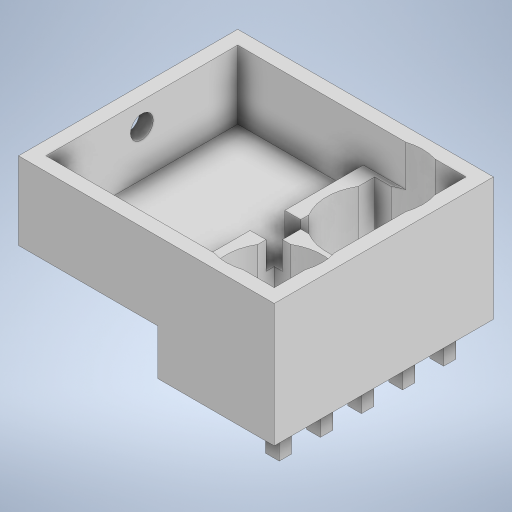
# Autodesk Inventor part: Suporte Eletroimã
Saved by Autodesk Inventor 2023 (Build 270158000, 158)
## iProperties
Created: 2023-03-07
Part Number: Suporte Eletroimã
Material: Genérico
Document SubType Name: Modeling
Designer: Inteli
Density: 1 g/cm^3
Appearance: Padrão
Author: Inteli
## iProperties of the stored document Suporte Eletroimã_3DPrint.ipt
Created: 2023-03-09
Part Number: Suporte Eletroimã_3DPrint
Material: Genérico
Document SubType Name: Modeling
Designer: Inteli
Density: 1 g/cm^3
Appearance: Padrão
Author: Inteli
Autodesk Inventor part; units mm, degrees
ref_plane "YZ Plane" through (0, 0, 0) normal (1, 0, 0) x (0, 1, 0)
ref_plane "XZ Plane" through (0, 0, 0) normal (0, 1, 0) x (-1, 0, 0)
ref_plane "XY Plane" through (0, 0, 0) normal (0, 0, 1) x (1, 0, 0)
sketch "Esboço1" plane through (0, 0, 0) normal (0, 1, 0) x (-1, 0, 0)
  circle A0 centre (0, 11) radius 10.5
  circle A1 centre (0, -11) radius 10.5
  line L0 (9, 2) -> (-9, 2)
  line L1 (-9, -2) -> (9, -2)
  line L2 (9, 20) -> (-9, 20)
  line L3 (-9, -20) -> (9, -20)
  line L4 (43, 24) -> (-13, 24)
  line L5 (-13, 24) -> (-13, -24)
  line L6 (-13, -24) -> (43, -24)
  line L7 (43, -24) -> (43, 24)
  line L8 (9, -20) -> (9, -2)
  line L9 (9, 2) -> (9, 20)
  line L10 (-9, 20) -> (-9, 2)
  line L11 (-9, -2) -> (-9, -20)
  point P0 (-9, 5.5917)
  point P1 (-9, 16.4083)
  point P2 (-5.4083, 20)
  point P3 (5.4083, 20)
  point P4 (9, 16.4083)
  point P5 (9, 5.5917)
  point P6 (5.4083, 2)
  point P7 (-5.4083, 2)
  point P8 (-9, -5.5917)
  point P9 (-5.4083, -2)
  point P10 (5.4083, -2)
  point P11 (9, -5.5917)
  point P12 (9, -16.4083)
  point P13 (5.4083, -20)
  point P14 (-5.4083, -20)
  point P15 (-9, -16.4083)
  point P16 (0, 0)
  point P17 (0, 21.5)
  point P18 (0, 21.5)
  point P19 (0, -21.5)
  point P20 (0, -21.5)
  dimension "d93" = 21
  dimension "d94" = 21
  dimension "d16" = 40
  dimension "d17" = 18
  dimension "d18" = 56
  dimension "d61" = 48
  dimension "d62" = 22
  constraints: 24 end point, 6 parallel, 3 coincident, 2 horizontal, 2 perpendicular, 1 vertical, 6 other
  measures "d16" distance of L3.start L2.end
  measures "d17" distance of L3.start L3.end
  measures "d18" distance of L6.end L5.end
  measures "d61" distance of L4.end L5.end
  measures "d62" distance of point (0, 11) point (0, -11)
extrude "Base Principal dos Imãs" add sketch "Esboço1" along normal blind 25
sketch "Esboço9" plane through (0, 0, 0) normal (0, -1, 0) x (1, 0, 0)
  line L0 (-43, 24) -> (13, 24) projected
  line L1 (13, -24) -> (-43, -24) projected
  line L2 (13, 24) -> (-43, 24)
  line L3 (-43, 24) -> (-43, -24)
  line L4 (-43, -24) -> (13, -24)
  line L5 (13, -24) -> (13, 24)
  point P0 (0, 0)
  point P1 (-43, 24)
  point P2 (13, -24)
  constraints: 8 end point, 2 parallel, 1 horizontal, 1 perpendicular
extrude "Fundo" add sketch "Esboço9" along normal blind 2
sketch "Esboço13" plane through (0, 25, 0) normal (0, 1, 0) x (1, 0, 0)
  line L0 (10, 21) -> (-40, 21)
  line L1 (-40, 21) -> (-40, -21)
  line L2 (-40, -21) -> (10, -21)
  line L3 (10, -21) -> (10, 21)
  line L4 (10, 21) -> (-40, -21) construction
  line L5 (-40, 21) -> (10, -21) construction
  line L6 (13, 24) -> (-43, 24) projected
  point P0 (0, 0)
  point P1 (0, 0)
  point P2 (25, 0)
  point P3 (10, 0)
  dimension "d84" = 50
  constraints: 12 end point, 1 coincident, 1 horizontal, 1 vertical
  measures "d84" distance of L2.end L1.end
extrude "PCB / Tampa" cut sketch "Esboço13" against normal blind 9
sketch "Esboço14" plane through (0, 25, 0) normal (0, 1, 0) x (1, 0, 0)
  line L0 (-9, -2) -> (-5.4083, -2) projected
  line L1 (-7.2042, -2) -> (-9, -3.7958)
  line L2 (-9, -5.5917) -> (-9, -2) projected
  line L3 (-7.2042, -2) -> (-7.2042, 2)
  line L4 (-9, 2) -> (-5.4083, 2) projected
  line L5 (-9, 2) -> (-9, 5.5917) projected
  line L6 (-9, 3.7958) -> (-7.2042, 2)
  line L7 (-9, -3.7958) -> (-12.5, -3.7958)
  line L8 (-12.5, -3.7958) -> (-12.5, 3.7958)
  line L9 (-12.5, 3.7958) -> (-9, 3.7958)
  point P0 (0, 0)
  dimension "d183" = 3.5
  constraints: 12 end point, 4 midpoint, 3 perpendicular, 1 horizontal
  measures "d183" distance of L1.end L7.end
extrude "Espaço Fio (Validar)" cut sketch "Esboço14" against normal blind 15
sketch "Esboço16" plane through (0, -2, 0) normal (0, -1, 0) x (1, 0, 0)
  line L0 (13, 24) -> (-43, 24) projected
  line L1 (-43, -24) -> (13, -24) projected
  line L2 (13, -24) -> (13, 24) projected
  line L3 (9.4436, 19.35) -> (6.4436, 19.35)
  line L4 (6.4436, 19.35) -> (6.4436, 16.65)
  line L5 (6.4436, 16.65) -> (9.4436, 16.65)
  line L6 (9.4436, 16.65) -> (9.4436, 19.35)
  line L7 (9.4436, 19.35) -> (6.4436, 16.65) construction
  line L8 (6.4436, 19.35) -> (9.4436, 16.65) construction
  line L9 (9.4436, 10.35) -> (6.4436, 10.35)
  line L10 (6.4436, 10.35) -> (6.4436, 7.65)
  line L11 (6.4436, 7.65) -> (9.4436, 7.65)
  line L12 (9.4436, 7.65) -> (9.4436, 10.35)
  line L13 (9.4436, 10.35) -> (6.4436, 7.65) construction
  line L14 (6.4436, 10.35) -> (9.4436, 7.65) construction
  line L15 (9.4436, 1.35) -> (6.4436, 1.35)
  line L16 (6.4436, 1.35) -> (6.4436, -1.35)
  line L17 (6.4436, -1.35) -> (9.4436, -1.35)
  line L18 (9.4436, -1.35) -> (9.4436, 1.35)
  line L19 (9.4436, 1.35) -> (6.4436, -1.35) construction
  line L20 (6.4436, 1.35) -> (9.4436, -1.35) construction
  line L21 (9.4436, -7.65) -> (6.4436, -7.65)
  line L22 (6.4436, -7.65) -> (6.4436, -10.35)
  line L23 (6.4436, -10.35) -> (9.4436, -10.35)
  line L24 (9.4436, -10.35) -> (9.4436, -7.65)
  line L25 (9.4436, -7.65) -> (6.4436, -10.35) construction
  line L26 (6.4436, -7.65) -> (9.4436, -10.35) construction
  line L27 (9.4436, -16.65) -> (6.4436, -16.65)
  line L28 (6.4436, -16.65) -> (6.4436, -19.35)
  line L29 (6.4436, -19.35) -> (9.4436, -19.35)
  line L30 (9.4436, -19.35) -> (9.4436, -16.65)
  line L31 (9.4436, -16.65) -> (6.4436, -19.35) construction
  line L32 (6.4436, -16.65) -> (9.4436, -19.35) construction
  point P0 (0, 0)
  point P1 (7.9436, 18)
  point P2 (7.9436, 9)
  point P3 (7.9436, 0)
  point P4 (7.9436, -9)
  point P5 (7.9436, -18)
  dimension "d132" = 9
  dimension "d144" = 9
  constraints: 60 end point, 2 midpoint, 2 parallel, 2 vertical, 1 horizontal, 1 perpendicular, 44 other
  measures "d144" distance of L3.start L9.start
sketch "Esboço17" plane through (-43, 25, -24) normal (-1, 0, 0) x (0, 0, 1)
  line L0 (0, -27) -> (0, 0) projected
  line L1 (48, -27) -> (48, 0) projected
  line L2 (0, 0) -> (48, 0)
  line L3 (48, 0) -> (48, -3)
  line L4 (48, -3) -> (0, -3)
  line L5 (0, -3) -> (0, 0)
  point P0 (24, -25)
  point P1 (0, -3)
  dimension "d109" = 3
  constraints: 8 end point, 2 parallel, 1 horizontal, 1 perpendicular, 1 point on line
  measures "d109" distance of L2.end L3.end
sketch "Esboço19" plane through (-43, -2, -24) normal (-1, 0, 0) x (0, 0, 1)
  line L0 (48, 0) -> (0, 0) projected
  line L1 (17.5, 20) -> (28.5, 20)
  line L2 (28.5, 20) -> (28.5, 12)
  line L3 (28.5, 12) -> (17.5, 12)
  line L4 (17.5, 12) -> (17.5, 20)
  line L5 (0, 24) -> (46, 24) projected
  point P0 (24, 2)
  dimension "d123" = 11
  dimension "d124" = 8
  constraints: 8 end point, 2 parallel, 1 horizontal, 1 perpendicular
  measures "d123" distance of L2.end L3.end
  measures "d124" distance of L1.end L2.end
extrude "Extrusão19" add sketch "Esboço16" along normal blind 7
fillet "Arredondamento da face2" radius 1 1 edges at (6.4436, -2, 18)
fillet "Arredondamento da face3" radius 1 2 edges at (5.9436, -2, 19.35) (7.9436, -2, 19.35)
fillet "Arredondamento da face4" radius 1 2 edges at (9.4436, -2, 19.85) (9.4436, -2, 18)
fillet "Arredondamento da face5" radius 1 3 edges at (9.9436, -2, 16.65) (7.9436, -2, 16.65) (5.9436, -2, 16.65)
fillet "Arredondamento da face6" radius 1 1 edges at (9.4436, -2, 9)
fillet "Arredondamento da face7" radius 1 2 edges at (9.9436, -2, 10.35) (7.9436, -2, 10.35)
fillet "Arredondamento da face8" radius 1 1 edges at (6.4436, -2, 9.5)
fillet "Arredondamento da face9" radius 1 2 edges at (5.9436, -2, 7.65) (8.4436, -2, 7.65)
fillet "Arredondamento da face10" radius 1 1 edges at (6.4436, -2, 0)
fillet "Arredondamento da face11" radius 1 2 edges at (5.9436, -2, -1.35) (7.9436, -2, -1.35)
fillet "Arredondamento da face12" radius 1 2 edges at (7.9436, -2, 1.35) (5.9436, -2, 1.35)
fillet "Arredondamento da face13" radius 1 3 edges at (9.4436, -2, 1.85) (9.4436, -2, 0) (9.4436, -2, -1.85)
fillet "Arredondamento da face14" radius 1 1 edges at (9.4436, -2, -9)
fillet "Arredondamento da face15" radius 1 2 edges at (9.9436, -2, -7.65) (7.9436, -2, -7.65)
fillet "Arredondamento da face16" radius 1 2 edges at (6.4436, -2, -7.15) (6.4436, -2, -9)
fillet "Arredondamento da face17" radius 1 3 edges at (9.9436, -2, -10.35) (7.9436, -2, -10.35) (5.9436, -2, -10.35)
fillet "Arredondamento da face18" radius 1 1 edges at (7.9436, -2, -19.35)
fillet "Arredondamento da face19" radius 1 2 edges at (9.4436, -2, -19.85) (9.4436, -2, -18)
fillet "Arredondamento da face20" radius 1 2 edges at (6.4436, -2, -19.85) (6.4436, -2, -18)
fillet "Arredondamento da face21" radius 1 3 edges at (5.9436, -2, -16.65) (7.9436, -2, -16.65) (9.9436, -2, -16.65)
sketch "Esboço21" plane through (0, -2, 0) normal (0, -1, 0) x (1, 0, 0)
  arc A0 (-9, -5.5917) -> (-9, -16.4083) centre (0, -11) ccw projected
  line L0 (13, 24) -> (-43, 24) projected
  line L1 (-43, 24) -> (-43, -24)
  line L2 (-43, -24) -> (-12.5, -24)
  line L3 (-12.5, -24) -> (-12.5, -11)
  line L4 (-12.5, -11) -> (-12.5, 24)
  line L5 (-43, -24) -> (13, -24) projected
  line L6 (-12.5, 24) -> (-43, 24)
  line L7 (-43, 24) -> (-43, -24) projected
  point P0 (0, 0)
  constraints: 10 end point, 2 point on line, 1 collinear, 1 perpendicular
extrude "Rebaixo Externo" cut sketch "Esboço21" against normal blind 10
sketch "Esboço22" plane through (0, 16, 0) normal (0, 1, 0) x (1, 0, 0)
  line L0 (-12.5, -24) -> (-12.5, 24) projected
  line L1 (-40, 21) -> (-3.2016, 21) projected
  line L2 (-12.5, 21) -> (-40, 21)
  line L3 (-40, -21) -> (-40, 21) projected
  line L4 (-40, 21) -> (-40, -21)
  line L5 (-40, -21) -> (-12.5, -21)
  line L6 (-12.5, -21) -> (-12.5, 21)
  point P0 (0, 0)
  point P1 (-12.5, 21)
  constraints: 8 end point, 2 collinear, 2 perpendicular, 1 point on line
extrude "Espaço Fios" cut sketch "Esboço22" against normal blind 6
sketch "Esboço23" plane through (-40, 25, 21) normal (1, 0, 0) x (0, 0, -1)
  circle A0 centre (21, -5) radius 2.5 projected
  circle A1 centre (21, -5) radius 2.5
  constraints: 1 centre point, 1 coincident
extrude "Furo" cut sketch "Esboço23" against normal up to surface (3 mm away)
